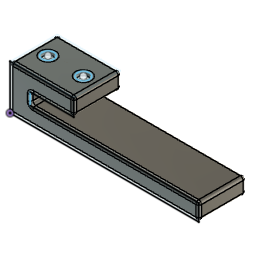
HX711 Test Jig v1 (Autodesk Fusion 360 design; units mm, degrees)
Autodesk Fusion 360 part; units mm, degrees
sketch "Sketch1" plane through (0, 0, 0) normal (0, 1, 0) x (1, 0, 0)
  line L0 (0, 0) -> (0, -19)
  line L1 (0, -19) -> (27, -19)
  line L2 (27, -19) -> (27, -12)
  line L3 (27, -12) -> (8.5117, -12)
  line L4 (8.5117, -12) -> (8.5117, -7)
  line L5 (8.5117, -7) -> (80, -7)
  line L6 (80, -7) -> (80, 0)
  line L7 (80, 0) -> (0, 0)
  dimension "d1" = 80
  dimension "d2" = 27
  dimension "d3" = 5
  dimension "d4" = 7
  dimension "d5" = 7
  constraint coincident L0.start L7.end
  constraint vertical L0
  constraint perpendicular L0 L1
  constraint perpendicular L1 L2
  constraint perpendicular L2 L3
  constraint perpendicular L3 L4
  constraint perpendicular L4 L5
  constraint perpendicular L5 L6
  constraint perpendicular L0 L7
  measures "d1" distance of L0.start L6.end
  measures "d2" distance of L0 L2
  measures "d3" distance of L3 L5
  measures "d4" distance of L1 L3
  measures "d5" distance of L5 L7
extrude "Extrude1" add sketch "Sketch1" along normal blind 20
sketch "Sketch2" plane through (0, 0, 19) normal (0, 0, 1) x (-1, 0, 0)
  line L0 (0, 0) -> (-27, 0)
  line L1 (-27, 0) -> (-27, -20)
  line L2 (-27, -20) -> (0, -20)
  line L3 (0, -20) -> (0, 0)
  circle A0 centre (-6, -10.0712) radius 2.5
  circle A1 centre (-21, -10.0712) radius 2.5
  dimension "d8" = 15
  dimension "d9" = 5
  dimension "d10" = 5
  dimension "d11" = 6
  measures "d8" distance of A0.centre A1.centre
  measures "d9" diameter of A0
  measures "d10" diameter of A1
  measures "d11" distance of L3 A0.centre
hole "Hole1" at (6, 10.0712, 19) direction (0, 0, -1) diameter 4.234 depth 10 tip angle 118
thread "Thread1" "ISO Metric profile 5.0 M5x0.8 6H"
hole "Hole2" at (21, 10.0712, 19) direction (0, 0, -1) diameter 4.234 depth 10 tip angle 118
thread "Thread2" "ISO Metric profile 5.0 M5x0.8 6H"
fillet "Fillet1" radius 1.2 9 faces at (32.3411, 6.6667, 7) (2.8372, 20, 10.3333) (53.3333, 6.6667, 0) (80, 13.3333, 4.6667) (2.8372, 0, 10.3333) (15.6938, 2.7213, 19) (27, 13.3333, 16.6667) (11.9708, 9.971, 12) (0, 6.6667, 6.3333)
